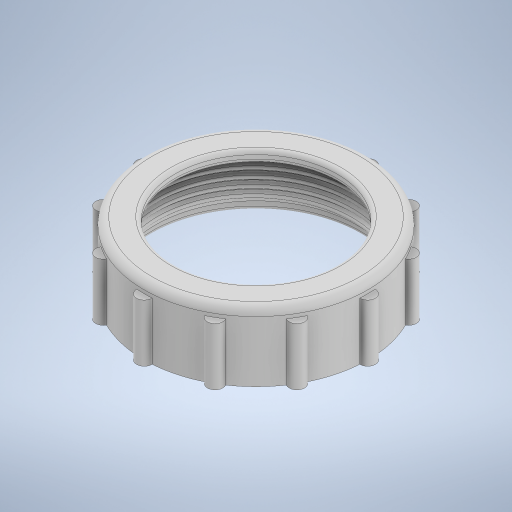
# Autodesk Inventor part: Rebreather-HoseRetainer
Saved by Autodesk Inventor 2023 (Build 270158000, 158)
## iProperties
Created: 2022-11-09
Part Number: Rebreather-HoseRetainer
Material: Generic
Document SubType Name: Modeling
Designer: incep
Density: 1 g/cm^3
Appearance: Default
Author: incep
## iProperties of the stored document Rebreather-HoseRetainer_3DPrint.ipt
Created: 2022-11-09
Part Number: Rebreather-HoseRetainer_3DPrint
Material: Generic
Document SubType Name: Modeling
Designer: incep
Density: 1 g/cm^3
Appearance: Default
Author: incep
Autodesk Inventor part; units mm, degrees
ref_plane "YZ Plane" through (0, 0, 0) normal (1, 0, 0) x (0, 1, 0)
ref_plane "XZ Plane" through (0, 0, 0) normal (0, 1, 0) x (-1, 0, 0)
ref_plane "XY Plane" through (0, 0, 0) normal (0, 0, 1) x (1, 0, 0)
sketch "Sketch1" plane through (0, 0, 0) normal (0, 0, 1) x (1, 0, 0)
  line L0 (-26.25, 0) -> (26.25, 0) construction
  line L1 (26.25, 0) -> (26.25, -14.9) construction
  line L2 (26.25, -14.9) -> (-26.25, -14.9) construction
  line L3 (-26.25, -14.9) -> (-26.25, 0) construction
  line L4 (-29.25, 3) -> (29.25, 3) construction
  line L5 (29.25, 3) -> (29.25, -14.9)
  line L6 (29.25, -14.9) -> (-29.25, -14.9) construction
  line L7 (-29.25, -14.9) -> (-29.25, 3)
  line L8 (-29.25, -14.9) -> (-26.25, -14.9) construction
  line L9 (26.25, -14.9) -> (29.25, -14.9) construction
  line L10 (-27.25, -12) -> (27.25, -12) construction
  line L11 (27.25, -12) -> (27.25, -14.9)
  line L12 (27.25, -14.9) -> (-27.25, -14.9) construction
  line L13 (-27.25, -14.9) -> (-27.25, -12)
  line L14 (-29.25, -14.9) -> (-27.25, -14.9)
  line L15 (-26.25, -12) -> (-26.25, 0)
  line L16 (-27.25, -12) -> (-26.25, -12)
  line L17 (27.25, -12) -> (26.25, -12)
  line L18 (26.25, -12) -> (26.25, 0)
  line L19 (-21.25, 3) -> (21.25, 3) construction
  line L20 (21.25, 3) -> (21.25, 0)
  line L21 (21.25, 0) -> (-21.25, 0) construction
  line L22 (-21.25, 0) -> (-21.25, 3)
  line L23 (-29.25, 3) -> (-21.25, 3)
  line L24 (21.25, 3) -> (29.25, 3)
  line L25 (27.25, -14.9) -> (29.25, -14.9)
  line L26 (21.25, 0) -> (26.25, 0)
  line L27 (24.6767, -10.1833) -> (26.25, -10.1833) construction
  line L28 (26.25, -10.1833) -> (26.25, -12) construction
  line L29 (26.25, -12) -> (24.6767, -12) construction
  line L30 (24.6767, -12) -> (24.6767, -10.1833) construction
  line L31 (26.25, -12) -> (24.6767, -11.0917) construction
  line L32 (24.6767, -11.0917) -> (26.25, -10.1833) construction
  line L33 (-25.2, 0) -> (25.2, 0) construction
  line L34 (25.2, 0) -> (25.2, -12) construction
  line L35 (25.2, -12) -> (-25.2, -12) construction
  line L36 (-25.2, -12) -> (-25.2, 0) construction
  arc A0 (25.4616, -10.6385) -> (25.4616, -11.5448) centre (25.7233, -11.0917) ccw construction
  arc A1 (25.4616, -10.6385) -> (25.4616, -11.5448) centre (25.7233, -11.0917) ccw
  line L37 (26.25, -10.1833) -> (25.4616, -10.6385)
  line L38 (25.4616, -11.5448) -> (26.25, -12)
  line L39 (26.25, -10.1833) -> (26.25, -12)
  line L40 (0, -18.48) -> (0, 6.58) projected
  point P0 (0, 0)
  point P1 (0, 0)
  point P2 (0, 3)
  point P3 (0, 3)
  point P4 (0, -12)
  point P5 (0, 0)
  point P6 (0, 0)
  dimension "d0" = 14.9
  dimension "d1" = 52.5
  dimension "d2" = 3
  dimension "d3" = 3
  dimension "d4" = 54.5
  dimension "d5" = 12
  dimension "d6" = 5
  dimension "d7" = 1.8167
  dimension "d8" = 60
  dimension "d9" = 50.4
  constraints: 80 end point, 15 collinear, 12 parallel, 9 perpendicular, 8 horizontal, 7 midpoint, 6 point on line, 5 coincident, 4 point on circle, 3 tangent, 2 centre point, 2 vertical alignment, 1 concentric, 1 horizontal alignment
  measures "d0" distance of L0.end L1.end
  measures "d1" distance between parallel lines of L1 L3
  measures "d2" distance between parallel lines of L1 L5
  measures "d3" distance between parallel lines of L0 L4
  measures "d4" distance between parallel lines of L11 L13
  measures "d5" distance between parallel lines of L0 L10
  measures "d6" distance between parallel lines of L1 L20
  measures "d7" distance of L27.end L28.end
  measures "d8" angle of L32 L31
  measures "d9" distance between parallel lines of L34 L36
coil "Coil1" sketch "Sketch1" operation add axis through (0, -10, 0) along (0, 1, 0) pitch 2.1167 turns 5.169291 hand right contours L38 A1 L37 L18
revolve "Revolution1" add sketch "Sketch1" angle 360 about axis through (0, -10, 0) along (0, 1, 0) contours L5 L25 L11 L17 L18 L26 L20 L24
sketch "Sketch2" plane through (0, -14.9, 0) normal (0, -1, 0) x (1, 0, 0)
  circle A0 centre (0, 0) radius 29.25 projected
  circle A1 centre (-29.25, 0) radius 2
  circle A2 centre (0, 0) radius 27.25 projected
  point P0 (-29.1816, -1.9988)
  point P1 (-29.1816, 1.9988)
  constraints: 1 centre point, 1 tangent, 2 other
extrude "Extrusion1" add sketch "Sketch2" against normal blind 15 contours A0 A1 picked at (-29.9065, 0.0821)
pattern_circular "Circular Pattern1" count 12 over 360 about axis through (0, -10, 0) along (0, 1, 0) of "Extrusion1"
fillet "Fillet1" radius 2 1 edges at (-29.25, 3, 0)
fillet "Fillet2" radius 1 3 edges at (-21.25, 3, 0) (-21.25, 0, 0) (-27.25, -14.9, 0)
body "Solid1"
